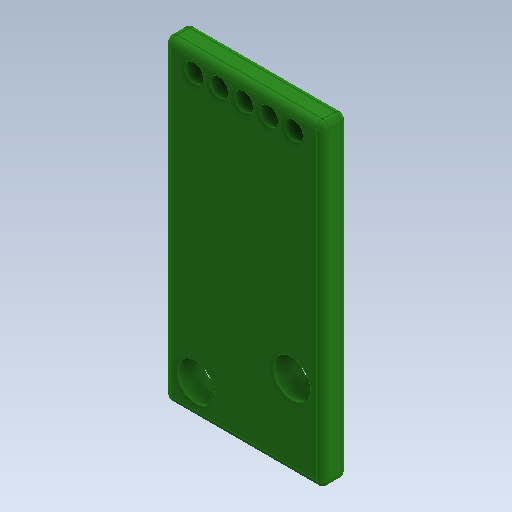
# Autodesk Inventor part: Czujnik AltIMU-10
Saved by Autodesk Inventor 2020 (Build 240168000, 168)
## iProperties
Created: 2021-10-10
Part Number: Czujnik AltIMU-10
Material: Ogólny
Document SubType Name: Modeling
Designer: Komputer
Density: 1 g/cm^3
Appearance: Domyślna
Mass: 0.590776 g
Surface Area: 8.01732 cm^2
Volume: 0.590776 cm^3
Author: Komputer
Autodesk Inventor part; units mm, degrees
ref_plane "YZ Plane" through (0, 0, 0) normal (1, 0, 0) x (0, 1, 0)
ref_plane "XZ Plane" through (0, 0, 0) normal (0, 1, 0) x (-1, 0, 0)
ref_plane "XY Plane" through (0, 0, 0) normal (0, 0, 1) x (1, 0, 0)
sketch "Szkic1" plane through (0, 0, 0) normal (0, 0, 1) x (1, 0, 0)
  line L0 (6.35, -12.7) -> (-6.35, -12.7)
  line L1 (-6.35, -12.7) -> (-6.35, 12.7)
  line L2 (-6.35, 12.7) -> (6.35, 12.7)
  line L3 (6.35, 12.7) -> (6.35, -12.7)
  line L4 (6.35, -12.7) -> (-6.35, 12.7) construction
  line L5 (-6.35, -12.7) -> (6.35, 12.7) construction
  point P0 (0, 0)
  dimension "d0" = 12.7
  dimension "d1" = 25.4
  constraints: 12 end point, 2 midpoint, 2 parallel, 1 horizontal, 1 perpendicular
  measures "d0" distance of L1.end L2.end
  measures "d1" distance of L0.end L1.end
extrude "Wyciągnięcie proste1" add sketch "Szkic1" along normal blind 2
fillet "Zaokrąglenie1" radius 0.5 12 edges at (0, 12.7, 2) (0, 12.7, 0) (-6.35, 12.7, 1) (6.35, 12.7, 1) (6.35, 0, 2) (6.35, 0, 0) (6.35, -12.7, 1) (0, -12.7, 2) (-6.35, 0, 2) (-6.35, -12.7, 1) (-6.35, 0, 0) (0, -12.7, 0)
sketch "Szkic2" plane through (0, 0, 0) normal (0, 0, -1) x (-1, 0, 0)
  line L0 (-5.85, -12.2) -> (5.85, -12.2) projected
  line L1 (-5.85, -12.2) -> (-5.85, -6.1)
  line L2 (-5.85, 12.2) -> (-5.85, -12.2) projected
  line L3 (-5.85, -6.1) -> (-3.85, -6.1)
  line L4 (5.85, -12.2) -> (5.85, 12.2) projected
  line L5 (5.85, -12.2) -> (3.85, -12.2)
  line L6 (3.85, -12.2) -> (3.85, -10.2)
  circle A0 centre (-3.85, -6.1) radius 1.5
  circle A1 centre (3.85, -10.2) radius 1.5
  line L7 (5.85, 12.2) -> (-5.85, 12.2) projected
  line L8 (-5.85, 12.2) -> (-5.85, 11.2)
  line L9 (0, 12.2) -> (0, 11.2)
  line L10 (0, 11.2) -> (-2, 11.2)
  line L11 (-2, 11.2) -> (-4, 11.2)
  line L12 (0, 11.2) -> (2, 11.2)
  line L13 (2, 11.2) -> (4, 11.2)
  circle A2 centre (-4, 11.2) radius 0.75
  circle A3 centre (-2, 11.2) radius 0.75
  circle A4 centre (0, 11.2) radius 0.75
  circle A5 centre (2, 11.2) radius 0.75
  circle A6 centre (4, 11.2) radius 0.75
  point P0 (0, 0)
  dimension "d5" = 6.1
  dimension "d8" = 2
  dimension "d9" = 2
  dimension "d10" = 2
  dimension "d11" = 3
  dimension "d12" = 3
  dimension "d13" = 1
  dimension "d14" = 1
  dimension "d15" = 2
  dimension "d16" = 2
  dimension "d17" = 2
  dimension "d18" = 2
  dimension "d19" = 1.5
  dimension "d20" = 1.5
  dimension "d21" = 1.5
  dimension "d22" = 1.5
  dimension "d23" = 1.5
  constraints: 20 end point, 7 centre point, 7 coincident, 4 point on line, 3 perpendicular, 1 horizontal, 1 midpoint, 1 vertical
  measures "d5" distance of L0.start L1.end
  measures "d8" distance of L1.end L3.end
  measures "d9" distance of L0.end L5.end
  measures "d10" distance of L5.end L6.end
  measures "d11" diameter of A0
  measures "d12" diameter of A1
  measures "d13" distance of L2.start L8.end
  measures "d14" distance of L9.start L9.end
  measures "d15" distance of L9.end L10.end
  measures "d16" distance of L10.end L11.end
  measures "d17" distance of L9.end L12.end
  measures "d18" distance of L12.end L13.end
  measures "d19" diameter of A2
  measures "d20" diameter of A3
  measures "d21" diameter of A4
  measures "d22" diameter of A5
  measures "d23" diameter of A6
extrude "Wyciągnięcie proste2" cut sketch "Szkic2" against normal blind 2 contours A1 | A6 | A5 L13 L12 | L12 L13 A5 | A2 | A3 L11 L10 | L10 L11 A3 | A4 L12 L9 | L9 L10 A4 | A0 | L12 A4 L10
